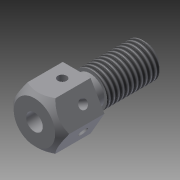
# Autodesk Inventor part: 13_5
Saved by Autodesk Inventor 2015 (Build 190159000, 159)
## iProperties
Created: 2015-03-31
Part Number: 13_5
Material: Generic
Document SubType Name: Modeling
Designer: WASHHSST
Density: 1 g/cm^3
Appearance: Default
Author: WASHHSST
Autodesk Inventor part; units mm, degrees
ref_plane "YZ Plane" through (0, 0, 0) normal (1, 0, 0) x (0, 1, 0)
ref_plane "XZ Plane" through (0, 0, 0) normal (0, 1, 0) x (-1, 0, 0)
ref_plane "XY Plane" through (0, 0, 0) normal (0, 0, 1) x (1, 0, 0)
sketch "Sketch1" plane through (0, 0, 0) normal (0, 0, 1) x (1, 0, 0)
  line L0 (3.175, -5.4993) -> (-3.175, -5.4993)
  line L1 (-3.175, -5.4993) -> (-6.35, 0)
  line L2 (-6.35, 0) -> (-3.175, 5.4993)
  line L3 (-3.175, 5.4993) -> (3.175, 5.4993)
  line L4 (3.175, 5.4993) -> (6.35, 0)
  line L5 (6.35, 0) -> (3.175, -5.4993)
  circle A0 centre (0, 0) radius 6.35
  line L6 (-10.4606, 10.0968) -> (12.3681, 10.0968) construction
  dimension "d0" = 12.7
  constraints: 14 end point, 2 coincident, 1 horizontal, 1 parallel, 16 other
extrude "Extrusion1" add sketch "Sketch1" against normal blind 9.652 contours L0 L1 L2 L3 L4 L5
sketch "Sketch3" plane through (0, 0, 0) normal (0, 0, 1) x (1, 0, 0)
  point P0 (0, 0)
  point P1 (0, 0)
  constraints: 1 coincident
hole "Hole1" at (0, 0, 0) direction (0, 0, -1) diameter 3.81 depth 7.874
sketch "Sketch5" plane through (0, 0, -9.652) normal (0, 0, -1) x (-1, 0, 0)
  circle A0 centre (0, 0) radius 3.302
  dimension "d10" = 6.604
  constraints: 2 coincident, 1 centre point
  measures "d10" diameter of A0
extrude "Extrusion2" add sketch "Sketch5" along normal blind 3.048
sketch "Sketch6" plane through (0, 0, -12.7) normal (0, 0, -1) x (-1, 0, 0)
  circle A0 centre (0, 0) radius 3.937
  dimension "d13" = 7.874
  constraints: 1 centre point, 1 coincident
  measures "d13" diameter of A0
extrude "Extrusion3" add sketch "Sketch6" along normal blind 12.7
chamfer "Chamfer1" distance 0.762 angle 45 1 edges at (3.937, 0, -25.4) measured on face at (1.2987, -0.8702, -25.4)
thread "Thread1" size "5/16-24 UNF" class "3A" standard "ANSI Unified Screw Threads" full length
sketch "Sketch7" plane through (-3.175, 5.4993, 0) normal (0, 1, 0) x (1, 0, 0)
  line L0 (0, 0) -> (0, 9.652) projected
  line L1 (0, 6.35) -> (6.35, 6.35)
  line L2 (6.35, 0) -> (6.35, 9.652) projected
  line L3 (-0.762, 12.7) -> (7.112, 12.7) projected
  point P0 (3.175, 0)
  point P1 (3.175, 6.35)
  dimension "d21" = 6.35
  dimension "d22" = 6.35
  dimension "d23" = 3.175
  constraints: 2 end point, 2 point on line, 1 horizontal, 1 midpoint
  measures "d21" distance between parallel lines of L1 L3
  measures "d22" distance between parallel lines of L2 L0
  measures "d23" distance from line of point (3.175, 6.35) L0
hole "Hole2" at (0, 5.4993, -6.35) direction (0, -1, 0) diameter 2.032 depth 6.35
pattern_circular "Circular Pattern1" count 6 over 360 about axis through (0, 0, -3.937) along (0, 0, 1) of "Hole2"
sketch "Sketch13" plane through (0, 0, 0) normal (0, 0, 1) x (1, 0, 0)
  circle A0 centre (0, 0) radius 5.4993
  line L0 (-3.175, 5.4993) -> (3.175, 5.4993) projected
  circle A1 centre (0, 0) radius 4.7373
  dimension "d42" = 0.762
  constraints: 2 centre point, 1 coincident, 1 tangent
  measures "d42" radial gap between concentric circles of A0 A1
extrude "Extrusion4" cut sketch "Sketch13" against normal blind 25.4 draft 45 contours A1 keep common part
body "Solid1"
